OdriveBracket_v4 (Autodesk Fusion 360 design; units mm, degrees)
Autodesk Fusion 360 part; units mm, degrees
note: some values were not read from the file. Set by a fixed rule: which sketch regions a step uses.
sketch "Sketch1" plane through (0, 0, 0) normal (0, 0, 1) x (1, 0, 0)
  line L0 (0, 0) -> (64.8, 0)
  line L1 (64.8, 0) -> (64.8, -4.8432)
  line L2 (64.8, -4.8432) -> (0, -4.8432)
  line L3 (0, -4.8432) -> (0, 0)
  line L4 (0, -4.8432) -> (-5, -4.8432)
  line L5 (-5, -4.8432) -> (-5, 50.1568)
  line L6 (-5, 50.1568) -> (0, 50.1568)
  line L7 (0, 50.1568) -> (0, -4.8432)
  line L8 (64.8, -4.8432) -> (69.8, -4.8432)
  line L9 (69.8, -4.8432) -> (69.8, 50.1568)
  line L10 (69.8, 50.1568) -> (64.8, 50.1568)
  line L11 (64.8, 50.1568) -> (64.8, -4.8432)
  line L12 (64.8, 42.25) -> (64.8, 39.75)
  circle A0 centre (64.8, 41) radius 1
  circle A1 centre (0, 44) radius 1.25
  dimension "d1" = 64.8
  dimension "d2" = 5
  dimension "d3" = 5
  dimension "d4" = 55
  dimension "d5" = 55
  dimension "d6" = 2.5
  dimension "d7" = 2
  dimension "d8" = 2.5
  dimension "d31" = 44
  dimension "d34" = 41
  constraint horizontal L0
  constraint vertical L1
  constraint horizontal L2
  constraint vertical L3
  constraint coincident L0.start L3.end
  constraint horizontal L4
  constraint vertical L5
  constraint horizontal L6
  constraint vertical L7
  constraint horizontal L8
  constraint vertical L9
  constraint horizontal L10
  constraint vertical L11
  constraint coincident L11 L12.start
  constraint parallel L11 L12
  constraint midpoint L12 A0.centre
  constraint coincident L7 A1.centre
  measures "d1" distance of L0.start L0.end
  measures "d2" distance of L2.end L4.end
  measures "d3" distance of L1.end L8.end
  measures "d4" distance of L1.end L10.end
  measures "d5" distance of L4.end L5.end
  measures "d6" distance of L12.start L12.end
  measures "d7" diameter of A0
  measures "d8" diameter of A1
  measures "d31" distance of L0 A1.centre
  measures "d34" distance of L0 A0.centre
extrude "Extrude1" add sketch "Sketch1" along normal blind 1
sketch "Sketch2" plane through (0, 0, 1) normal (0, 0, 1) x (-1, 0, 0)
  line L0 (0, 0) -> (0, -42.75)
  arc A0 (0, -42.75) -> (0, -45.25) centre (0, -44) ccw
  line L1 (0, -45.25) -> (0, -50.1568)
  line L2 (0, -50.1568) -> (5, -50.1568)
  line L3 (5, -50.1568) -> (5, 4.8432)
  line L4 (5, 4.8432) -> (-69.8, 4.8432)
  line L5 (-69.8, 4.8432) -> (-69.8, -50.1568)
  line L6 (-69.8, -50.1568) -> (-64.8, -50.1568)
  line L7 (-64.8, -50.1568) -> (-64.8, -42)
  arc A1 (-64.8, -42) -> (-64.8, -40) centre (-64.8, -41) ccw
  line L8 (-64.8, -40) -> (-64.8, 0)
  line L9 (-64.8, 0) -> (0, 0)
  line L10 (5, -50.1568) -> (-2.5, -50.1568)
  line L11 (-2.5, -50.1568) -> (-2.5, -30.1568)
  line L12 (-2.5, -30.1568) -> (5, -30.1568)
  line L13 (5, -30.1568) -> (5, -50.1568)
  line L14 (-69.8, -50.1568) -> (-62.3, -50.1568)
  line L15 (-62.3, -50.1568) -> (-62.3, -30.1568)
  line L16 (-62.3, -30.1568) -> (-69.8, -30.1568)
  line L17 (-69.8, -30.1568) -> (-69.8, -50.1568)
  line L18 (5, 4.8432) -> (-69.8, 4.8432)
  line L19 (-69.8, 4.8432) -> (-69.8, -1.6568)
  line L20 (-69.8, -1.6568) -> (5, -1.6568)
  line L21 (5, -1.6568) -> (5, 4.8432)
  dimension "d11" = 7.5
  dimension "d12" = 20
  dimension "d13" = 7.5
  dimension "d14" = 20
  dimension "d25" = 6.5
  constraint horizontal L10
  constraint vertical L11
  constraint horizontal L12
  constraint vertical L13
  constraint coincident L2.end L3.start
  constraint horizontal L14
  constraint vertical L15
  constraint horizontal L16
  constraint vertical L17
  constraint coincident L5.end L6.start
  constraint horizontal L18
  constraint vertical L19
  constraint horizontal L20
  constraint vertical L21
  constraint coincident L5 L19.end
  constraint coincident L3.end L4.start
  measures "d11" distance of L2.end L10.end
  measures "d12" distance of L2.end L12.end
  measures "d13" distance of L5.end L14.end
  measures "d14" distance of L5.end L16.end
  measures "d25" distance of L18 L20
extrude "Extrude2" [suppressed]
fillet "Fillet1" [suppressed]
fillet "Fillet2" [suppressed]
fillet "Fillet3" [suppressed]
fillet "Fillet4" [suppressed]
fillet "Fillet5" [suppressed]
mirror "Mirror1" [suppressed]
equation "d1 = 64.3 mm + 0.5 mm"
equation "d2 = d3"
equation "d5 = d4"
equation "d11 = d13"
equation "d14 = d12"
equation "d31 = 42 mm + 2 mm"
equation "d34 = 39 mm + 2 mm"
